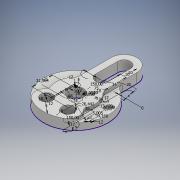
# Autodesk Inventor part: лаб,2_2
Saved by Autodesk Inventor 2018 (Build 220112000, 112)
## iProperties
Created: 2020-04-08
Part Number: лаб,2_2
Material: Типовые
Document SubType Name: Modeling
Designer: Nikita
Density: 1 g/cm^3
Appearance: По умолчанию
Author: Nikita
Autodesk Inventor part; units mm, degrees
ref_plane "YZ Plane" through (0, 0, 0) normal (1, 0, 0) x (0, 1, 0)
ref_plane "XZ Plane" through (0, 0, 0) normal (0, 1, 0) x (-1, 0, 0)
ref_plane "XY Plane" through (0, 0, 0) normal (0, 0, 1) x (1, 0, 0)
sketch "Эскиз1" plane through (0, 0, 0) normal (0, 0, 1) x (1, 0, 0)
  arc A0 (-25, 43.3013) -> (25, 43.3013) centre (0, 0) ccw
  circle A1 centre (0, 0) radius 12
  line L0 (-50, 0) -> (50, 0) construction
  line L1 (0, 0) -> (-24.9984, -43.3022) construction
  line L2 (0, 0) -> (25.0049, -43.3022) construction
  circle A2 centre (0, 0) radius 33 construction
  circle A3 centre (-16.499, -28.5794) radius 9
  circle A4 centre (16.4989, -28.5795) radius 9
  arc A5 (-28.5669, -16.606) -> (-28.0784, -10.5643) centre (-33.4841, -13.1678) ccw
  arc A6 (-26.1975, -14.6174) -> (-26.1978, -14.6176) centre (-16.499, -28.5794) ccw
  arc A7 (-28.5357, -16.5745) -> (-24.9984, -43.3022) centre (-16.499, -28.5794) ccw
  line L3 (0, 0) -> (0, 75)
  arc A8 (20, 75) -> (-20, 75) centre (0, 75) ccw
  arc A9 (10, 75) -> (-10, 75) centre (0, 75) ccw
  line L4 (0, 75) -> (0, 41)
  arc A10 (-20, 41) -> (20, 41) centre (0, 41) ccw construction
  arc A11 (-10, 41) -> (10, 41) centre (0, 41) ccw
  line L5 (-10, 75) -> (-10, 41)
  line L6 (10, 75) -> (10, 41)
  line L7 (0, 21) -> (-26, 21) construction
  line L8 (0, 21) -> (26, 21) construction
  line L9 (-28.0784, -10.5643) -> (28.0784, -10.5643) construction
  arc A12 (28.0091, -10.7467) -> (29.5474, -17.6828) centre (33.4989, -13.1678) ccw
  arc A13 (-0.4419, -29.9967) -> (0.0837, -32.9999) centre (16.4989, -28.5795) ccw
  arc A14 (24.9984, -43.3022) -> (28.5357, -16.5746) centre (16.4989, -28.5795) ccw
  arc A15 (-25, 43.3013) -> (-20, 51.9615) centre (-30, 51.9615) ccw
  arc A16 (20, 51.9615) -> (25, 43.3013) centre (30, 51.9615) ccw
  arc A17 (20, 24.8998) -> (21.6667, 20.7498) centre (26, 24.8998) ccw
  arc A18 (-21.6667, 20.7498) -> (-20, 24.8998) centre (-26, 24.8998) ccw
  arc A19 (-21.4243, 21) -> (-27.753, -11.3916) centre (0, 0) ccw
  arc A20 (27.8299, -11.2025) -> (21.4243, 21) centre (0, 0) ccw
  arc A21 (-24.9984, -43.3022) -> (24.9984, -43.3022) centre (0, 0) ccw
  line L10 (-20, 75) -> (-20, 51.9615)
  line L11 (20, 75) -> (20, 51.9615)
  line L12 (20, 51.9615) -> (20, 24.8998)
  line L13 (-20, 51.9615) -> (-20, 24.8998)
  dimension "d0" = 100
  dimension "d1" = 24
  dimension "d2" = 66
  dimension "d3" = 18
  dimension "d4" = 18
  dimension "d7" = 12
  dimension "d10" = 75
  dimension "d11" = 20
  dimension "d12" = 10
  dimension "d13" = 34
  dimension "d14" = 20
  dimension "d15" = 10
  dimension "d24" = 26
  dimension "d25" = 26
  dimension "d29" = 12
  dimension "d30" = 20
  dimension "d31" = 20
  dimension "d32" = 17
  dimension "d37" = 21
  dimension "d38" = 31.5643
  dimension "d40" = 34.1678
  dimension "d66" = 12
  dimension "d67" = 12
  dimension "d68" = 30
  dimension "d69" = 30
  dimension "d70" = 30.004
  dimension "d71" = 150.002
  dimension "d72" = 13.4989
  dimension "d73" = 9.5474
  dimension "d74" = 8.0784
  dimension "d75" = 8.0091
  dimension "d76" = 5.0049
  dimension "d77" = 0
  dimension "d78" = 20.4419
  dimension "d79" = 46.1975
  dimension "d80" = 46.1978
  dimension "d81" = 47.753
  dimension "d82" = 48.0784
  constraints: 52 point on circle, 28 end point, 22 centre point, 16 tangent, 11 coincident, 5 vertical, 4 horizontal, 4 point on line, 2 parallel
  measures "d0" diameter of A0
  measures "d1" diameter of A1
  measures "d2" diameter of A2
  measures "d3" diameter of A3
  measures "d4" diameter of A4
  measures "d7" diameter of A5
  measures "d10" distance of L3.start L3.end
  measures "d11" radius of A8
  measures "d12" radius of A9
  measures "d13" distance of L4.start L4.end
  measures "d14" radius of A10
  measures "d15" radius of A11
  measures "d24" distance of L7.start L7.end
  measures "d25" distance of L7.start L8.end
  measures "d29" diameter of A12
  measures "d30" diameter of A15
  measures "d31" diameter of A16
  measures "d32" radius of A14
  measures "d37" distance between parallel lines of L0 L8
  measures "d38" distance between parallel lines of L9 L8
  measures "d40" distance from line of A12.centre L8
  measures "d66" diameter of A17
  measures "d67" diameter of A18
  measures "d68" radius of A20
  measures "d69" radius of A19
  measures "d70" angle of L2 L11
  measures "d71" angle of L11 L1
  measures "d72" distance from line of A12.centre L11
  measures "d73" distance from line of A12.end L11
  measures "d74" distance from line of L9.end L11
  measures "d75" distance from line of A12.start L11
  measures "d76" distance from line of L2.end L11
  measures "d77" distance from line of A10.end L11
  measures "d78" distance from line of A13.start L11
  measures "d79" distance from line of A6.start L11
  measures "d80" distance from line of A6.end L11
  measures "d81" distance from line of A19.end L11
  measures "d82" distance from line of L9.start L11
extrude "Выдавливание1" add sketch "Эскиз1" along normal blind 10 contours A15 L13 A18 A19 A5 A6 A0 | A14 A12 A20 A17 L12 A16 A0 | A12 A14
extrude "Выдавливание2" add sketch "Эскиз1" along normal blind 15 contours A6 A5 A19 A18 L13 L10 A8 L11 L12 A17 A20 A12 A14 A0 | A6 | A19 A5 | A12 A20
